Aluminium rod (Autodesk Fusion 360 design; units mm, degrees)
Autodesk Fusion 360 part; units mm, degrees
sketch "Sketch1" plane through (0, 0, 0) normal (0, 1, 0) x (1, 0, 0)
  circle A0 centre (0, 0) radius 2.95
  circle A1 centre (0, 0) radius 1.75
  dimension "d1" = 5.9
  dimension "d4" = 3.5
  constraint coincident A0.centre A1.centre
  measures "d1" diameter of A0
  measures "d4" diameter of A1
extrude "Extrude1" add sketch "Sketch1" along normal blind 220
